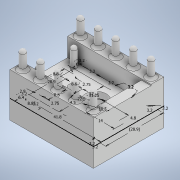
# Autodesk Inventor part: motor holder under
Saved by Autodesk Inventor 2022 (Build 260153000, 153)
## iProperties
Created: 2021-11-29
Part Number: motor holder under
Material: Generic
Document SubType Name: Modeling
Designer: Alec Warren
Density: 1 g/cm^3
Appearance: Default
Author: Alec Warren
Autodesk Inventor part; units mm, degrees
ref_plane "YZ Plane" through (0, 0, 0) normal (1, 0, 0) x (0, 1, 0)
ref_plane "XZ Plane" through (0, 0, 0) normal (0, 1, 0) x (-1, 0, 0)
ref_plane "XY Plane" through (0, 0, 0) normal (0, 0, 1) x (1, 0, 0)
sketch "Sketch1" plane through (0, 0, 0) normal (0, 1, 0) x (-1, 0, 0)
  line L0 (0, 0) -> (0, 22.5)
  line L1 (0, 22.5) -> (-41.8, 22.5)
  line L2 (-41.8, 22.5) -> (-41.8, 0)
  line L3 (-41.8, 0) -> (0, 0)
  line L4 (0, 11.25) -> (-37, 11.25)
  line L5 (-37, 11.25) -> (-41.8, 11.25)
  line L6 (-39.4, 11.25) -> (-25.4, 11.25)
  line L7 (-25.4, 11.25) -> (-14.15, 11.25)
  line L8 (-14.15, 11.25) -> (-5.55, 11.25)
  line L9 (-5.55, 11.25) -> (-5.55, 2.45)
  line L10 (-5.55, 11.25) -> (-5.55, 20.05)
  circle A0 centre (-5.55, 2.45) radius 1.375
  circle A1 centre (-5.55, 20.05) radius 1.375
  line L11 (-37, 0) -> (-37, 22.5)
  line L12 (0, 22.5) -> (0, 28.9)
  line L13 (0, 0) -> (0, -6.4)
  line L14 (0, -6.4) -> (-41.8, -6.4)
  line L15 (-41.8, -6.4) -> (-41.8, 0)
  line L16 (-41.8, 22.5) -> (-41.8, 28.9)
  line L17 (-41.8, 28.9) -> (0, 28.9)
  line L18 (0, -3.2) -> (-3.2, -3.2)
  line L19 (-41.8, -3.2) -> (-38.6, -3.2)
  line L20 (-41.8, 25.7) -> (-38.6, 25.7)
  line L21 (0, 25.7) -> (-3.2, 25.7)
  circle A2 centre (-3.2, -3.2) radius 1.6
  circle A3 centre (-38.6, -3.2) radius 1.6
  circle A4 centre (-38.6, 25.7) radius 1.6
  circle A5 centre (-3.2, 25.7) radius 1.6
  circle A6 centre (-25.4, 11.25) radius 5.25
  line L22 (-38.6, -3.2) -> (-3.2, -3.2)
  line L23 (-3.2, -3.2) -> (-20.9, -3.2)
  circle A7 centre (-12.05, -3.2) radius 1.6
  line L24 (-38.6, -3.2) -> (-20.9, -3.2)
  circle A8 centre (-20.9, -3.2) radius 1.6
  circle A9 centre (-29.75, -3.2) radius 1.6
  circle A10 centre (-3.2, 25.7) radius 1.6
  circle A11 centre (-38.6, 25.7) radius 1.6
  circle A12 centre (-12.05, 25.7) radius 1.6
  circle A13 centre (-20.9, 25.7) radius 1.6
  circle A14 centre (-29.75, 25.7) radius 1.6
  circle A15 centre (-14.15, 11.25) radius 2.25
  circle A16 centre (-3.2, 25.7) radius 1.45
  line L25 (-41.8, 25.7) -> (-41.8, -3.2)
  circle A17 centre (-12.05, 25.7) radius 1.45
  circle A18 centre (-20.9, 25.7) radius 1.45
  circle A19 centre (-29.75, 25.7) radius 1.45
  circle A20 centre (-38.6, 25.7) radius 1.45
  circle A21 centre (-3.2, -3.2) radius 1.45
  circle A22 centre (-12.05, -3.2) radius 1.45
  circle A23 centre (-20.9, -3.2) radius 1.45
  circle A24 centre (-29.75, -3.2) radius 1.45
  circle A25 centre (-38.6, -3.2) radius 1.45
  dimension "d0" = 22.5
  dimension "d1" = 41.8
  dimension "d2" = 37
  dimension "d3" = 4.8
  dimension "d4" = 14
  dimension "d5" = 11.25
  dimension "d6" = 8.6
  dimension "d7" = 8.8
  dimension "d8" = 8.8
  dimension "d9" = 2.75
  dimension "d10" = 2.75
  dimension "d12" = 6.4
  dimension "d13" = 6.4
  dimension "d15" = 3.2
  dimension "d16" = 3.2
  dimension "d17" = 3.2
  dimension "d18" = 3.2
  dimension "d19" = 3.2
  dimension "d20" = 3.2
  dimension "d21" = 3.2
  dimension "d22" = 3.2
  dimension "d23" = 10.5
  dimension "d24" = 3.2
  dimension "d25" = 3.2
  dimension "d26" = 3.2
  dimension "d35" = 4.5
  dimension "d36" = 2.9
  dimension "d37" = 28.9
  dimension "d40" = 8.85
  dimension "d43" = 28.9
  constraints: 52 end point, 26 centre point, 10 coincident, 10 midpoint, 8 horizontal, 7 perpendicular, 6 point on line, 6 vertical, 5 symmetric about line, 1 collinear, 23 other
  measures "d0" distance of L0.start L0.end
  measures "d1" distance of L0.end L1.end
  measures "d2" distance of L4.start L4.end
  measures "d3" distance of L4.end L5.end
  measures "d4" distance of L6.start L6.end
  measures "d5" distance of L6.end L7.end
  measures "d6" distance of L7.end L8.end
  measures "d7" distance of L8.end L9.end
  measures "d8" distance of L8.end L10.end
  measures "d9" diameter of A0
  measures "d10" diameter of A1
  measures "d12" distance of L0.end L12.end
  measures "d13" distance of L0.start L13.end
  measures "d15" distance of L18.start L18.end
  measures "d16" distance of L19.start L19.end
  measures "d17" distance of L20.start L20.end
  measures "d18" distance of L21.start L21.end
  measures "d19" diameter of A2
  measures "d20" diameter of A3
  measures "d21" diameter of A4
  measures "d22" diameter of A5
  measures "d23" diameter of A6
  measures "d24" diameter of A7
  measures "d25" diameter of A8
  measures "d26" diameter of A9
  measures "d35" diameter of A15
  measures "d36" diameter of A16
  measures "d37" distance of L20.start L19.start
  measures "d40" distance of A16.centre A17.centre
  measures "d43" distance of A16.centre A21.centre
extrude "Extrusion1" add sketch "Sketch1" along normal blind 3.2 contours L3 L11 L4 A6 A15 L0 | L13 L18 A2 L22 A7 A8 A9 A3 L19 L15 L3 | L4 A15 A6 L11 L1 L0 | L3 L2 L5 L11 | L13 L14 L15 L19 A3 L22 A9 A8 A7 A2 L18 | L1 L16 L17 L12 | L5 L2 L1 L11 | A2 L22 A21 L18 | L18 A21 L22 A2 | A21 L22 L18 | L18 L22 A21 | A3 L22 A25 L19 | L19 A25 L22 A3 | A7 L22 A22 | L22 A22 A7 | A25 L22 L19 | L19 L22 A25 | A22 L22 | L22 A22 | A9 L22 A24 | L22 A24 A9 | A8 L22 A23 | L22 A23 A8 | A24 L22 | L22 A24 | A23 L22 | L22 A23 | A0 | A1 | A4 | A5 | A12 | A13 | A14 | A16 | A17 | A18 | A19 | A20
extrude "Extrusion2" add sketch "Sketch1" along normal blind 9.3 from surface at 3.2 contours L13 L18 A2 L22 A7 A8 A9 A3 L19 L15 L3 | L13 L14 L15 L19 A3 L22 A9 A8 A7 A2 L18 | L1 L16 L17 L12 | A2 L22 A21 L18 | L18 A21 L22 A2 | A21 L22 L18 | L18 L22 A21 | A3 L22 A25 L19 | L19 A25 L22 A3 | A7 L22 A22 | L22 A22 A7 | A25 L22 L19 | L19 L22 A25 | A22 L22 | L22 A22 | A9 L22 A24 | L22 A24 A9 | A8 L22 A23 | L22 A23 A8 | A24 L22 | L22 A24 | A23 L22 | L22 A23 | A0 | A1 | A4 | A5 | A12 | A13 | A14 | A16 | A17 | A18 | A19 | A20
extrude "Extrusion4" add sketch "Sketch1" along normal blind 8.7 from surface at 3.2 contours L3 L2 L5 L11 | L5 L2 L1 L11
extrude "Extrusion5" add sketch "Sketch1" along normal blind 9 from surface at 12.5 contours A21 L22 L18 | L18 L22 A21 | A25 L22 L19 | L19 L22 A25 | A22 L22 | L22 A22 | A24 L22 | L22 A24 | A23 L22 | L22 A23 | A16 | A17 | A18 | A19 | A20
fillet "Fillet1" radius 1.45 10 edges at (4.65, 21.5, 25.7) (13.5, 21.5, 25.7) (22.35, 21.5, 25.7) (31.2, 21.5, 25.7) (40.05, 21.5, 25.7) (40.05, 21.5, -3.2) (31.2, 21.5, -3.2) (13.5, 21.5, -3.2) (4.65, 21.5, -3.2) (22.35, 21.5, -3.2)
fillet "Fillet2" radius 1.35 2 edges at (6.925, 12.5, 2.45) (6.925, 12.5, 20.05)
fillet "Fillet3" radius 1.2 10 edges at (4.65, 12.5, 25.7) (13.5, 12.5, 25.7) (4.65, 12.5, -3.2) (13.5, 12.5, -3.2) (22.35, 12.5, -3.2) (31.2, 12.5, -3.2) (40.05, 12.5, -3.2) (40.05, 12.5, 25.7) (31.2, 12.5, 25.7) (22.35, 12.5, 25.7)
extrude "Extrusion6" add sketch "Sketch1" against normal blind 9.5 contours L3 L11 L4 A6 A15 L0 | L13 L18 A2 L22 A7 A8 A9 A3 L19 L15 L3 | L4 A15 A6 L11 L1 L0 | L3 L2 L5 L11 | L13 L14 L15 L19 A3 L22 A9 A8 A7 A2 L18 | L1 L16 L17 L12 | L5 L2 L1 L11 | A2 L22 A21 L18 | L18 A21 L22 A2 | A15 L4 | L4 A15 | A21 L22 L18 | L18 L22 A21 | A3 L22 A25 L19 | L19 A25 L22 A3 | A7 L22 A22 | L22 A22 A7 | A25 L22 L19 | L19 L22 A25 | A22 L22 | L22 A22 | A9 L22 A24 | L22 A24 A9 | A8 L22 A23 | L22 A23 A8 | A24 L22 | L22 A24 | A23 L22 | L22 A23 | A0 | A1 | A4 | A5 | A12 | A13 | A14 | A16 | A17 | A18 | A19 | A20
body "Solid1"
